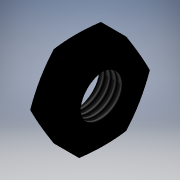
# Autodesk Inventor part: NT-03_CQS
Saved by Autodesk Inventor 2017.3 (Build 213256000, 256)
## iProperties
Part Number: NT-03_CQS
Material: Generic
Catalog Web Link: www.cadenas.de
Description: CQS/CDQS NUT-Compact Cylinder:Standard Type Double Acting,Single Rod
Vendor: SMC
Document SubType Name: Modeling
Designer: partserver
Manufacturer: SMC
Mass: 1.13131 g
Surface Area: 8.66514 cm^2
Volume: 1.13131 cm^3
Density: 1 g/cm^3
Appearance: PSOLRGB-0-0-0
Category: PARTsolutions
Company: SMC
Title: NT-03
Author: Cadenas PARTsolutions
Comments: Compact Cylinder:Standard Type Double Acting,Single Rod
PSOL_IDENT_0: {$CADENAS_DATA\23d-libs\smc_jp\actuator\compact_cylinder\cqs\cqs\parts\cqs_nut.prj},160 {VTYP=3D},{N
PSOL_IDENT_1: B=NT-03_CQS},{LINA=NT-03},{NN=CQS/CDQS NUT},{DATE=29.10.2021 06:14:24},{GEOMDATE=25.06.2018 02:28:00
PSOL_IDENT_2: },{VERSION=},{LINEID=40},{WBVAR=},{WBNUMERIC=}  {NB=NT-03_CQS},{LINA=NT-03},{KT=DUMMY},{BORE=25},{MO
PSOL_IDENT_3: DEL=NT-03},{B1=17},{H1=6},{MM=M10x1.25},{MMRA=10},{MMRP=1.25}
NB: NT-03_CQS
NN: CQS/CDQS NUT
NT: Compact Cylinder:Standard Type Double Acting,Single Rod
NBSYN: $MODEL._CQS
LINA: NT-03
CATALOG: SMC (JP
BORE: 25
MODEL: NT-03
B1: 17
H1: 6
MM: M10x1.25
SUPPLIER: SMC
ARTICLENO: NT-03_CQS
BOMINFO: NT-03
CREATOR: CADENAS GmbH
Autodesk Inventor part; units mm, degrees
sketch "Sketch_1" plane through (0, 0, 0) normal (0, 0, 1) x (1, 0, 0)
  line L0 (3, 0) -> (-3, 0)
  line L1 (-3, 8.5) -> (-3, 5)
  line L2 (-3, 5) -> (-2.3235, 4.3235)
  line L3 (-2.3235, 4.3235) -> (2.3235, 4.3235)
  line L4 (2.3235, 4.3235) -> (3, 5)
  line L5 (3, 5) -> (3, 8.5)
  line L6 (3, 8.5) -> (1.6335, 13.6)
  line L7 (1.6335, 13.6) -> (-1.6335, 13.6)
  line L8 (-1.6335, 13.6) -> (-3, 8.5)
  constraints: 18 end point
revolve "Revolution1" add sketch "Sketch_1" angle 360 about axis through (3, 0, 0) along (1, 0, 0)
thread "Thread1" size "M10x1.25" class "6H" standard "ISO Metric profile" full length
sketch "Sketch_2" plane through (0, 0, 0) normal (1, 0, 0) x (0, 1, 0)
  circle A0 centre (0, 0) radius 17
  line L0 (-4.9075, 8.5) -> (-9.815, 0)
  line L1 (-9.815, 0) -> (-4.9075, -8.5)
  line L2 (-4.9075, -8.5) -> (4.9075, -8.5)
  line L3 (4.9075, -8.5) -> (9.815, 0)
  line L4 (9.815, 0) -> (4.9075, 8.5)
  line L5 (4.9075, 8.5) -> (-4.9075, 8.5)
  constraints: 12 end point, 1 centre point
extrude "Extrusion1" cut sketch "Sketch_2" along normal mid plane 12
ref_plane "NUT_ROD_XY" through (0, 0, 0) normal (1, 0, 0) x (0, 0, -1)
ref_plane "NUT_ROD_YZ" through (0, 0, 0) normal (0, 0, -1) x (0, 1, 0)
ref_plane "NUT_ROD_ZX" through (0, 0, 0) normal (0, 1, 0) x (1, 0, 0)
body "Solid1"
